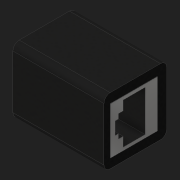
# Autodesk Inventor part: Ethernet Port
Saved by Autodesk Inventor 2017 SP1 (Build 210196100, 196)
## iProperties
Created: 2017-09-20
Part Number: Ethernet Port
Material: ABS Plastic
Document SubType Name: Modeling
Designer: Zach
Density: 1.06 g/cm^3
Appearance: Black
Author: Zach
Autodesk Inventor part; units mm, degrees
ref_plane "YZ Plane" through (0, 0, 0) normal (1, 0, 0) x (0, 1, 0)
ref_plane "XZ Plane" through (0, 0, 0) normal (0, 1, 0) x (-1, 0, 0)
ref_plane "XY Plane" through (0, 0, 0) normal (0, 0, 1) x (1, 0, 0)
sketch "Sketch1" plane through (0, 0, 0) normal (0, 0, 1) x (1, 0, 0)
  line L0 (0, 0) -> (29, 0)
  line L1 (29, 0) -> (29, 21)
  line L2 (29, 21) -> (0, 21)
  line L3 (0, 21) -> (0, 0)
  dimension "d0" = 29
  dimension "d1" = 21
  constraints: 8 end point, 2 parallel, 1 horizontal, 1 perpendicular
  measures "d0" distance of L2.end L1.end
  measures "d1" distance of L1.end L0.end
extrude "Extrusion1" add sketch "Sketch1" along normal blind 20
sketch "Sketch2" plane through (29, 0, 0) normal (1, 0, 0) x (0, 0, -1)
  line L0 (-7, 4) -> (-14, 4)
  line L1 (-14, 4) -> (-14, 17)
  line L2 (-14, 17) -> (-7, 17)
  line L3 (-7, 17) -> (-7, 4)
  line L4 (-20, 0) -> (-20, 21) construction
  line L5 (-14, 7) -> (-15.5, 7)
  line L6 (-15.5, 7) -> (-15.5, 14)
  line L7 (-15.5, 14) -> (-14, 14)
  line L8 (-14, 14) -> (-14, 7)
  line L9 (-15.5, 17) -> (-7, 17)
  line L10 (0, 21) -> (-20, 21) construction
  line L11 (-15.5, 12.5) -> (-16.5, 12.5)
  line L12 (-16.5, 12.5) -> (-16.5, 8.5)
  line L13 (-16.5, 8.5) -> (-15.5, 8.5)
  line L14 (-15.5, 8.5) -> (-15.5, 12.5)
  line L15 (0, 0) -> (0, 21) projected
  point P0 (-14, 10.5)
  point P1 (-20, 10.5)
  point P2 (-11.25, 17)
  point P3 (-10, 21)
  point P4 (-15.5, 10.5)
  dimension "d4" = 7
  dimension "d5" = 13
  dimension "d6" = 1.5
  dimension "d7" = 7
  dimension "d12" = 4
  dimension "d13" = 1
  dimension "d14" = 7
  constraints: 26 end point, 7 midpoint, 6 parallel, 4 horizontal, 3 perpendicular, 2 horizontal alignment, 2 point on line, 1 vertical alignment
  measures "d4" distance of L1.end L2.end
  measures "d5" distance of L0.end L1.end
  measures "d6" distance of L6.end L7.end
  measures "d7" distance of L5.end L6.end
  measures "d12" distance of L11.end L12.end
  measures "d13" distance of L11.start L11.end
  measures "d14" distance between parallel lines of L15 L3
extrude "Extrusion2" cut sketch "Sketch2" against normal blind 12.7
sketch "Sketch3" plane through (0, 0, 0) normal (-1, 0, 0) x (0, 0, 1)
  line L0 (14, 14) -> (14, 17) projected
  line L1 (15.5, 14) -> (14, 14) projected
  line L2 (15.5, 7) -> (15.5, 14) projected
  line L3 (14, 7) -> (15.5, 7) projected
  line L4 (7, 4) -> (14, 4) projected
  line L5 (7, 17) -> (7, 4) projected
  line L6 (14, 17) -> (7, 17) projected
  line L7 (14, 4) -> (14, 7) projected
  point P0 (0, 0)
extrude "Extrusion3" cut sketch "Sketch3" against normal blind 12.7
sketch "Sketch4" plane through (29, 0, 0) normal (1, 0, 0) x (0, 0, -1)
  line L0 (-18, 3) -> (-3, 3)
  line L1 (-3, 3) -> (-3, 18)
  line L2 (-3, 18) -> (-18, 18)
  line L3 (-18, 18) -> (-18, 3)
  line L4 (-20, 0) -> (-20, 21) projected
  line L5 (-15.5, 8.5) -> (-16.5, 8.5) projected
  line L6 (-15.5, 7) -> (-15.5, 8.5) projected
  line L7 (-14, 7) -> (-15.5, 7) projected
  line L8 (-14, 4) -> (-14, 7) projected
  line L9 (-7, 4) -> (-14, 4) projected
  line L10 (-7, 17) -> (-7, 4) projected
  line L11 (-14, 17) -> (-7, 17) projected
  line L12 (-14, 14) -> (-14, 17) projected
  line L13 (-15.5, 14) -> (-14, 14) projected
  line L14 (-15.5, 12.5) -> (-15.5, 14) projected
  line L15 (-16.5, 12.5) -> (-15.5, 12.5) projected
  line L16 (-16.5, 8.5) -> (-16.5, 12.5) projected
  point P0 (0, 0)
  point P1 (-18, 10.5)
  point P2 (-20, 10.5)
  dimension "d15" = 15
  dimension "d16" = 15
  dimension "d17" = 2
  constraints: 8 end point, 2 midpoint, 2 parallel, 1 horizontal, 1 horizontal alignment, 1 perpendicular
  measures "d15" distance of L0.end L1.end
  measures "d16" distance of L1.end L2.end
  measures "d17" distance between parallel lines of L4 L3
extrude "Extrusion4" add sketch "Sketch4" along normal blind 0.1
fillet "Fillet1" radius 2 4 edges at (14.5, 0, 0) (14.5, 0, 20) (14.5, 21, 20) (14.5, 21, 0)
body "Solid1"
